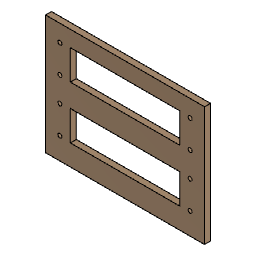
Connection box socket panel (Autodesk Fusion 360 design; units mm, degrees)
Autodesk Fusion 360 part; units mm, degrees
sketch "Sketch1" plane through (0, 0, 0) normal (0, 1, 0) x (1, 0, 0)
  line L0 (80, -60) -> (-80, -60)
  line L1 (-80, -60) -> (-80, 60)
  line L2 (-80, 60) -> (80, 60)
  line L3 (80, 60) -> (80, -60)
  line L4 (80, -60) -> (-80, 60) construction
  line L5 (-80, -60) -> (80, 60) construction
  line L6 (0, -60) -> (0, 60) construction
  line L7 (65.5, -15) -> (-65.5, -15) construction
  line L8 (-65.5, -15) -> (-65.5, -43) construction
  line L9 (-65.5, -43) -> (65.5, -43) construction
  line L10 (65.5, -43) -> (65.5, -15) construction
  line L11 (65.5, -15) -> (-65.5, -43) construction
  line L12 (-65.5, -15) -> (65.5, -43) construction
  line L13 (65.5, 10) -> (-65.5, 10) construction
  line L14 (-65.5, 10) -> (-65.5, 38) construction
  line L15 (-65.5, 38) -> (65.5, 38) construction
  line L16 (65.5, 38) -> (65.5, 10) construction
  line L17 (65.5, 10) -> (-65.5, 38) construction
  line L18 (-65.5, 10) -> (65.5, 38) construction
  circle A0 centre (65.5, -43) radius 2
  circle A1 centre (65.5, -15) radius 2
  circle A2 centre (-65.5, -43) radius 2
  circle A3 centre (-65.5, -15) radius 2
  circle A4 centre (-65.5, 10) radius 2
  circle A5 centre (-65.5, 38) radius 2
  circle A6 centre (65.5, 38) radius 2
  circle A7 centre (65.5, 10) radius 2
  line L19 (55, -44) -> (-55, -44)
  line L20 (-55, -44) -> (-55, -14)
  line L21 (-55, -14) -> (55, -14)
  line L22 (55, -14) -> (55, -44)
  line L23 (55, -44) -> (-55, -14) construction
  line L24 (-55, -44) -> (55, -14) construction
  line L25 (55, 9) -> (-55, 9)
  line L26 (-55, 9) -> (-55, 39)
  line L27 (-55, 39) -> (55, 39)
  line L28 (55, 39) -> (55, 9)
  line L29 (55, 9) -> (-55, 39) construction
  line L30 (-55, 9) -> (55, 39) construction
  point P0 (0, -29)
  point P1 (0, 24)
  point P2 (0, -29)
  point P3 (0, 24)
  dimension "d1" = 160
  dimension "d2" = 120
  dimension "d3" = 131
  dimension "d4" = 28
  dimension "d5" = 131
  dimension "d6" = 28
  dimension "d7" = 15
  dimension "d8" = 10
  dimension "d9" = 4
  dimension "d10" = 4
  dimension "d11" = 4
  dimension "d12" = 4
  dimension "d13" = 4
  dimension "d14" = 4
  dimension "d15" = 4
  dimension "d16" = 4
  dimension "d17" = 110
  dimension "d18" = 30
  dimension "d19" = 110
  dimension "d20" = 30
  constraint perpendicular L0 L1
  constraint parallel L0 L2
  constraint parallel L1 L3
  constraint horizontal L0
  constraint coincident L4 origin
  constraint coincident L5 origin
  constraint midpoint L0 L6.start
  constraint midpoint L2 L6.end
  constraint perpendicular L7 L8
  constraint parallel L7 L9
  constraint parallel L8 L10
  constraint horizontal L7
  constraint coincident L11 P2
  constraint coincident L12 P2
  constraint coincident L6 P2
  constraint perpendicular L13 L14
  constraint parallel L13 L15
  constraint parallel L14 L16
  constraint horizontal L13
  constraint coincident L17 P3
  constraint coincident L18 P3
  constraint coincident L6 P3
  constraint coincident L9.end L10.start
  constraint coincident L7.start L10.end
  constraint coincident L8.end L9.start
  constraint coincident L7.end L8.start
  constraint coincident L13.end L14.start
  constraint coincident L14.end L15.start
  constraint coincident L15.end L16.start
  constraint coincident L13.start L16.end
  constraint perpendicular L19 L20
  constraint parallel L19 L21
  constraint parallel L20 L22
  constraint horizontal L19
  constraint coincident L23 P2
  constraint coincident L24 P2
  constraint coincident P2 P0
  constraint perpendicular L25 L26
  constraint parallel L25 L27
  constraint parallel L26 L28
  constraint horizontal L25
  constraint coincident L29 P3
  constraint coincident L30 P3
  constraint coincident P3 P1
  measures "d1" distance of L1.end L2.end
  measures "d2" distance of L0.end L1.end
  measures "d3" distance of L8.end L9.end
  measures "d4" distance of L7.end L8.end
  measures "d5" distance of L14.end L15.end
  measures "d6" distance of L13.end L14.end
  measures "d7" distance of origin L7
  measures "d8" distance of origin L13
  measures "d9" diameter of A0
  measures "d10" diameter of A1
  measures "d11" diameter of A2
  measures "d12" diameter of A3
  measures "d13" diameter of A4
  measures "d14" diameter of A5
  measures "d15" diameter of A6
  measures "d16" diameter of A7
  measures "d17" distance of L20.end L21.end
  measures "d18" distance of L19.end L20.end
  measures "d19" distance of L26.end L27.end
  measures "d20" distance of L25.end L26.end
extrude "Extrude2" add sketch "Sketch1" along normal blind 6
extrude "Extrude1" [suppressed]
equation "d3 = 143 mm - 12 mm"
equation "d4 = 40 mm - 12 mm"
equation "d5 = 143 mm - 12 mm"
equation "d6 = 40 mm - 12 mm"
equation "d10 = d9"
equation "d11 = d9"
equation "d12 = d9"
equation "d13 = d9"
equation "d14 = d9"
equation "d15 = d9"
equation "d16 = d9"
named bodies: "Panel"
